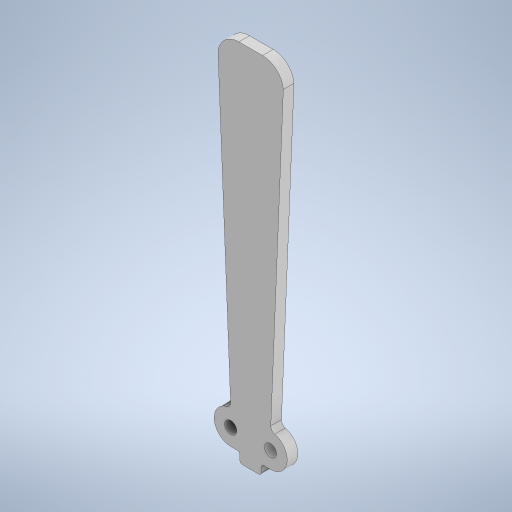
# Autodesk Inventor part: Blade
Saved by Autodesk Inventor 2023.5 (Build 275446000, 446)
## iProperties
Created: 2025-04-03
Part Number: Blade
Material: Generic
Document SubType Name: Modeling
Designer: huy20
Density: 1 g/cm^3
Appearance: Default
Author: huy20
Autodesk Inventor part; units mm, degrees
ref_plane "YZ Plane" through (0, 0, 0) normal (1, 0, 0) x (0, 1, 0)
ref_plane "XZ Plane" through (0, 0, 0) normal (0, 1, 0) x (-1, 0, 0)
ref_plane "XY Plane" through (0, 0, 0) normal (0, 0, 1) x (1, 0, 0)
sketch "Sketch1" plane through (0, 0, 0) normal (0, 0, 1) x (1, 0, 0)
  line L0 (12.4954, 128.3185) -> (7.6936, 14.3066)
  circle A0 centre (-7.62, 6.2119) radius 2.286
  line L1 (7.62, 8.4979) -> (7.9776, 8.4697)
  line L2 (7.2624, 3.954) -> (7.62, 3.9259)
  circle A1 centre (7.62, 6.2119) radius 2.286
  line L3 (-10.2607, 11.9867) -> (-10.7886, 11.7148)
  arc A2 (-9.1979, 12.3627) -> (-7.62, -0.1381) centre (-7.62, 6.2119) ccw
  arc A3 (7.62, -0.1381) -> (9.198, 12.3626) centre (7.62, 6.2119) ccw
  line L4 (-7.6934, 14.3065) -> (-12.4926, 128.3185)
  arc A4 (-4.1275, -2.9481) -> (-3.1275, -3.9481) centre (-3.1275, -2.9481) ccw
  arc A5 (3.1275, -3.9481) -> (4.1275, -2.9481) centre (3.1275, -2.9481) ccw
  line L5 (7.62, -0.1381) -> (5.1275, -0.1381)
  line L6 (-5.1275, -0.1381) -> (-7.62, -0.1381)
  arc A6 (-4.1275, -1.1381) -> (-5.1275, -0.1381) centre (-5.1275, -1.1381) ccw
  arc A7 (5.1275, -0.1381) -> (4.1275, -1.1381) centre (5.1275, -1.1381) ccw
  arc A8 (7.6968, 14.3841) -> (9.198, 12.3626) centre (9.6951, 14.2999) ccw
  arc A9 (-9.1979, 12.3627) -> (-7.6966, 14.3841) centre (-9.6949, 14.3) ccw
  line L7 (12.4954, 128.3185) -> (12.4954, 135.5817)
  line L8 (12.4954, 135.5817) -> (-12.4926, 135.5817)
  line L9 (-12.4926, 135.5817) -> (-12.4926, 128.3185)
  line L10 (-4.1275, -1.1381) -> (-4.1275, -2.9481)
  line L11 (-3.1275, -3.9481) -> (3.1275, -3.9481)
  line L12 (4.1275, -1.1381) -> (4.1275, -2.9481)
  point P0 (-5.1275, -0.1381)
  point P1 (0.0014, 135.5817)
  point P2 (0, 0)
  point P3 (-10.7886, 11.7148)
  dimension "d2" = 15.24
  dimension "d7" = 4
  dimension "d15" = 4.572
  dimension "d16" = 24.988
  dimension "d17" = 4.822
  dimension "d74" = 10.16
  dimension "d75" = 3.9482
  dimension "d76" = 6.35
  dimension "d77" = 1
  dimension "d78" = 177.588
  dimension "d79" = 92.088
  dimension "d80" = 92.412
  dimension "d81" = 119.665
  dimension "d82" = 8.3679
  dimension "d83" = 16.6229
  dimension "d84" = 4.5579
  dimension "d85" = 135.7199
  dimension "d86" = 7.0847
  dimension "d87" = 12.4954
  dimension "d88" = 9.0695
  dimension "d89" = 7.0849
  dimension "d90" = 15.3547
  dimension "d91" = 0
  dimension "d92" = 0.5294
  dimension "d93" = 4.8018
  dimension "d94" = 0.1709
  dimension "d95" = 0.3633
  dimension "d96" = 0.0048
  dimension "d97" = 2.913
  dimension "d98" = 10.0433
  dimension "d99" = 15.3733
  dimension "d100" = 18.3567
  dimension "d101" = 24.9658
  constraints: 26 end point, 19 point on circle, 15 tangent, 10 centre point, 6 equal radius, 6 point on line, 4 parallel, 3 coincident, 2 horizontal, 2 vertical, 1 collinear, 1 midpoint
  measures "d2" distance of A1.centre point (-7.62, 6.212)
  measures "d7" diameter of A9
  measures "d15" diameter of A0
  measures "d16" distance of L7.end L8.end
  measures "d17" angle of L4 L0
  measures "d74" distance from line of L11 A1.centre
  measures "d75" distance from line of L11 point (0, 0)
  measures "d76" radius of A3
  measures "d77" radius of A7
  measures "d78" angle of L0 L7
  measures "d79" angle of L1 L0
  measures "d80" angle of L0 L6
  measures "d81" angle of L3 L0
  measures "d82" distance between parallel lines of L12 L7
  measures "d83" distance between parallel lines of L10 L7
  measures "d84" distance between parallel lines of L1 L2
  measures "d85" distance between parallel lines of L8 L5
  measures "d86" distance from line of point (0, 0) L0
  measures "d87" distance from line of point (0, 0) L7
  measures "d88" distance from line of point (0, 0) L1
  measures "d89" distance from line of point (0, 0) L4
  measures "d90" distance from line of point (0, 0) L3
  measures "d91" distance from line of L7.start L0
  measures "d92" distance from line of L1.end L0
  measures "d93" distance from line of L0.end L7
  measures "d94" distance from line of L1.start L0
  measures "d95" distance from line of L2.end L0
  measures "d96" distance from line of L2.start L0
  measures "d97" distance from line of A7.end L0
  measures "d98" distance from line of A4.end L0
  measures "d99" distance from line of L4.start L0
  measures "d100" distance from line of L3.end L0
  measures "d101" distance from line of L9.end L0
extrude "Extrusion1" add sketch "Sketch1" along normal mid plane 4.077 contours L0 A8 A3 L5 A7 L12 A5 L11 A4 L10 A6 L6 A2 L3 A9 L4 L9 L8 L7
fillet "Fillet1" radius 8 2 edges at (12.4954, 135.5817, 0) (-12.4926, 135.5817, 0)
body "Solid1"
